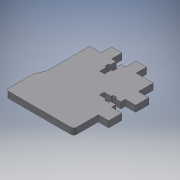
# Autodesk Inventor part: A8-0001
Saved by Autodesk Inventor 2016 SP2 (Build 200236200, 236)
## iProperties
Created: 2017-04-22
Part Number: A8-0001
Material: Generic
Document SubType Name: Modeling
Designer: EV
Density: 1 g/cm^3
Appearance: Default
Author: EV
Autodesk Inventor part; units mm, degrees
ref_plane "YZ Plane" through (0, 0, 0) normal (1, 0, 0) x (0, 1, 0)
ref_plane "XY Plane" through (0, 0, 0) normal (0, 0, 1) x (1, 0, 0)
sketch "Sketch1" plane through (0, 0, 0) normal (0, 1, 0) x (-1, 0, 0)
  line L0 (0, 0) -> (-49, 0)
  line L1 (-49, 0) -> (-49, -17.75)
  line L2 (-49, -17.75) -> (-56.5, -17.75)
  line L3 (-56.5, -17.75) -> (-56.5, -27.25)
  line L4 (-56.5, -27.25) -> (-49, -27.25)
  line L5 (-49, -27.25) -> (-49, -30.5)
  line L6 (-49, -30.5) -> (-45, -30.5)
  line L7 (-45, -30.5) -> (-45, -29.25)
  line L8 (-45, -29.25) -> (-42, -29.25)
  line L9 (-42, -29.25) -> (-42, -30.5)
  line L10 (-42, -30.5) -> (-37, -30.5)
  line L11 (-37, -30.5) -> (-37, -34)
  line L12 (-37, -34) -> (-42, -34)
  line L13 (-42, -34) -> (-42, -35.25)
  line L14 (-42, -35.25) -> (-45, -35.25)
  line L15 (-45, -35.25) -> (-45, -34)
  line L16 (-45, -34) -> (-49, -34)
  line L17 (-49, -34) -> (-49, -37.25)
  line L18 (-49, -37.25) -> (-56.5, -37.25)
  line L19 (-56.5, -37.25) -> (-56.5, -46.75)
  line L20 (-56.5, -46.75) -> (-49, -46.75)
  line L21 (-49, -46.75) -> (-49, -57.5)
  line L22 (-49, -57.5) -> (-36.55, -57.5)
  line L23 (-36.55, -57.5) -> (-36.55, -65)
  line L24 (-36.55, -65) -> (-29.05, -65)
  line L25 (-29.05, -65) -> (-29.05, -57.5)
  line L26 (-29.05, -57.5) -> (-25.675, -57.5)
  line L27 (-25.675, -57.5) -> (-25.675, -53.5)
  line L28 (-25.675, -53.5) -> (-26.925, -53.5)
  line L29 (-26.925, -53.5) -> (-26.925, -50.5)
  line L30 (-26.925, -50.5) -> (-25.675, -50.5)
  line L31 (-25.675, -50.5) -> (-25.675, -45.5)
  line L32 (-25.675, -45.5) -> (-22.175, -45.5)
  line L33 (-22.175, -45.5) -> (-22.175, -50.5)
  line L34 (-22.175, -50.5) -> (-20.925, -50.5)
  line L35 (-20.925, -50.5) -> (-20.925, -53.5)
  line L36 (-20.925, -53.5) -> (-22.175, -53.5)
  line L37 (-22.175, -53.5) -> (-22.175, -57.5)
  line L38 (-22.175, -57.5) -> (-18.8, -57.5)
  line L39 (-18.8, -57.5) -> (-18.8, -65)
  line L40 (-18.8, -65) -> (-11.3, -65)
  line L41 (-11.3, -65) -> (-11.3, -57.5)
  line L42 (-11.3, -57.5) -> (-3, -57.5)
  line L43 (-3, -57.5) -> (-3, -27.25)
  line L44 (-3, -27.25) -> (0, -19.5)
  line L45 (0, -19.5) -> (0, 0)
  dimension "d0" = 49
  dimension "d1" = 65
  dimension "d2" = 7.5
  dimension "d3" = 17.75
  dimension "d4" = 7.5
  dimension "d5" = 19.5
  dimension "d6" = 46
  dimension "d7" = 10
  dimension "d8" = 3.5
  dimension "d9" = 6
  dimension "d10" = 4
  dimension "d11" = 3
  dimension "d12" = 5
  dimension "d14" = 10.25
  dimension "d15" = 8.3
  dimension "d16" = 6
  dimension "d17" = 3.5
  dimension "d21" = 9.5
  constraints: 92 end point, 29 point on line, 28 perpendicular, 12 equal length, 1 horizontal, 1 parallel, 1 vertical
  measures "d0" distance of L0.start L0.end
  measures "d1" distance between parallel lines of L40 L0
  measures "d2" distance of L40.end L41.end
  measures "d3" distance between parallel lines of L2 L0
  measures "d4" distance of L39.end L40.end
  measures "d5" distance of L44.end L0.start
  measures "d6" distance between parallel lines of L1 L43
  measures "d7" distance between parallel lines of L18 L4
  measures "d8" distance between parallel lines of L16 L6
  measures "d9" distance between parallel lines of L14 L8
  measures "d10" distance of L5.end L6.end
  measures "d11" distance of L7.end L8.end
  measures "d12" distance of L9.end L10.end
  measures "d14" distance between parallel lines of L25 L39
  measures "d15" distance between parallel lines of L41 L43
  measures "d16" distance between parallel lines of L29 L35
  measures "d17" distance between parallel lines of L27 L37
  measures "d21" distance of L18.end L19.end
extrude "Extrusion1" add sketch "Sketch1" along normal blind 4.5
fillet "Fillet1" radius 2 4 edges at (0, 2.25, 0) (49, 2.25, 0) (0, 2.25, -19.5) (3, 2.25, -27.25)
ref_plane "Work Plane1" through (0, 2.25, 0) normal (0, 1, 0) x (-1, 0, 0)
equation "\"d16\" = d9"
equation "\"d17\" = d8"
equation "\"d22\" = 0.5 * THICKNESS"
equation "\"THICKNESS\" = 4.5"
body "Solid1"
